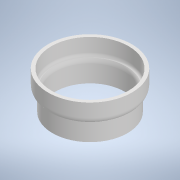
# Autodesk Inventor part: headset bearing
Saved by Autodesk Inventor 2022.2 (Build 262287010, 287A)
## iProperties
Created: 2022-04-06
Part Number: headset bearing
Material: Generic
Document SubType Name: Modeling
Designer: Finn Oriwohl
Density: 1 g/cm^3
Appearance: Default
Author: Finn Oriwohl
Autodesk Inventor part; units mm, degrees
ref_plane "YZ Plane" through (0, 0, 0) normal (1, 0, 0) x (0, 1, 0)
ref_plane "XZ Plane" through (0, 0, 0) normal (0, 1, 0) x (-1, 0, 0)
ref_plane "XY Plane" through (0, 0, 0) normal (0, 0, 1) x (1, 0, 0)
sketch "Sketch1" plane through (0, 0, 0) normal (0, 0, 1) x (1, 0, 0)
  line L0 (0, 0) -> (15, 0) construction
  line L1 (18, 3) -> (18, 9)
  line L2 (15, 0) -> (15, -7.7504)
  arc A0 (15, 0) -> (18, 3) centre (15, 3) ccw
  line L3 (15, 0) -> (15, 0)
  line L4 (16.5, 9) -> (16.5, 3)
  arc A1 (15, 1.5) -> (16.5, 3) centre (15, 3) ccw
  line L5 (15, 1.5) -> (0, 1.5)
  line L6 (13.5, -7.7504) -> (13.5, 0.8352)
  line L7 (13.5, 0.8352) -> (13.5, 0.1716)
  arc A2 (15, 1.5) -> (13.5, 0.8352) centre (15.2456, -1.0788) ccw
  line L8 (16.5, 9) -> (18, 9)
  line L9 (15, -7.7504) -> (13.5, -7.7504)
  line L10 (0, 0) -> (0, 2.7427)
  point P0 (18, 0)
  point P1 (13.5, 0.1716)
  dimension "d0" = 9
  dimension "d1" = 3
  dimension "d3" = 15
  dimension "d4" = 3
  dimension "d5" = 1.5
  dimension "d9" = 1.5
  constraints: 22 end point, 7 point on circle, 4 vertical, 3 centre point, 3 point on line, 2 horizontal, 2 tangent, 1 parallel, 3 other
  measures "d0" distance of point (18, 0) L1.end
  measures "d1" distance of L2.start point (18, 0)
  measures "d3" distance of L0.start L2.start
  measures "d4" radius of A0
  measures "d5" radial gap between concentric circles of A0 A1
  measures "d9" distance between parallel lines of L2 L6
revolve "Revolution1" add sketch "Sketch1" angle 360 about axis through (0, 0, 0) along (0, 1, 0)
equation "\"d9\" = d5"
body "Solid1"
